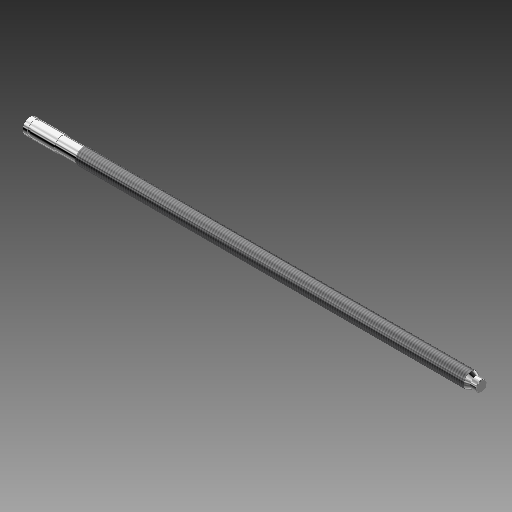
# Autodesk Inventor part: 201-05
Saved by Autodesk Inventor 2019 (Build 230136000, 136)
## iProperties
Company: Autodesk Inc.
Created: 2007-10-25
Part Number: 201-05
Document SubType Name: Modeling
Designer: Autodesk Inc.
Density: 8 g/cm^3
Mass: 244.897 g
Surface Area: 113.8 cm^2
Volume: 30.6121 cm^3
Material: Stainless Steel
Description: BALL SCREW SHAFT
Appearance: Chrome - Polished
Component Category: Lower Component
Author: Inventor
Autodesk Inventor part; units mm, degrees
ref_plane "YZ Plane" through (0, 0, 0) normal (1, 0, 0) x (0, 1, 0)
ref_plane "XZ Plane" through (0, 0, 0) normal (0, 1, 0) x (-1, 0, 0)
ref_plane "XY Plane" through (0, 0, 0) normal (0, 0, 1) x (1, 0, 0)
sketch "Sketch1" plane through (0, 0, 0) normal (0, 0, 1) x (1, 0, 0)
  line L0 (-64.9, 0) -> (389.4, 0) projected
  line L1 (0, 6.636) -> (0, -1.106) projected
  line L2 (0, 0) -> (0, 5.53)
  line L3 (0, 5.53) -> (3.25, 5.53)
  line L4 (3.25, 5.53) -> (3.25, 5.03)
  line L5 (3.25, 5.03) -> (5.25, 5.03)
  line L6 (5.25, 5.03) -> (5.25, 5.53)
  line L7 (5.25, 5.53) -> (22.75, 5.53)
  line L8 (22.75, 5.53) -> (22.75, 5.03)
  line L9 (22.75, 5.03) -> (37.75, 5.03)
  line L10 (37.75, 5.03) -> (37.75, 5.53)
  line L11 (37.75, 5.53) -> (320, 5.53)
  line L12 (320, 5.53) -> (320, 4)
  line L13 (320, 4) -> (324.5, 4)
  line L14 (324.5, 4) -> (324.5, 0)
  line L15 (0, 0) -> (324.5, 0)
  dimension "d0" = 37.75
  dimension "d1" = 15
  dimension "d2" = 17.5
  dimension "d3" = 2
  dimension "d4" = 11.06
  dimension "d5" = 0.5
  dimension "d6" = 0.5
  dimension "d7" = 320
  dimension "d8" = 324.5
  dimension "d9" = 8
  constraints: 28 end point, 7 parallel, 5 collinear, 3 perpendicular, 2 point on line
  measures "d0" distance between parallel lines of L10 L1
  measures "d1" distance between parallel lines of L10 L8
  measures "d2" distance of L6.end L7.end
  measures "d3" distance from line of L4 L5.end
  measures "d4" diameter of L11 L15
  measures "d5" distance between parallel lines of L7 L5
  measures "d6" distance between parallel lines of L7 L9
  measures "d7" distance between parallel lines of L2 L12
  measures "d8" distance between parallel lines of L2 L14
  measures "d9" diameter of L13 L15
revolve "Revolution1" add sketch "Sketch1" angle 360 about axis through (0, 0, 0) along (1, 0, 0)
chamfer "Chamfer1" distance 1.53 distance2 3 1 edges at (320, -5.53, 0) measured on face at (320, 4.9664, -0.4411)
chamfer "Chamfer2" distance 0.5 angle 45 1 edges at (324.5, -4, 0)
thread "Thread1" size "M12x1.75" class "6g" standard "ANSI Metric M Profile" full length
equation "\"d6\" = d5"
body "Solid1"
